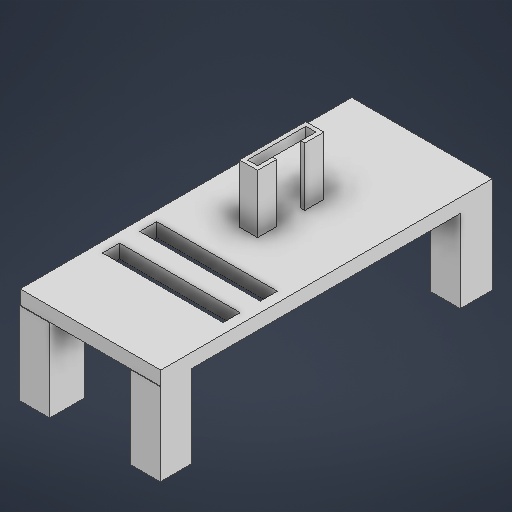
# Autodesk Inventor part: piano laterale
Saved by Autodesk Inventor 2026.2 (Build 302298000, 298)
## iProperties
Created: 2026-01-19
Part Number: piano laterale
Material: Generic
Document SubType Name: Modeling
Designer: ASUS
Density: 1 g/cm^3
Appearance: Default
Mass: 93.3252 g
Surface Area: 462.271 cm^2
Volume: 93.3252 cm^3
Author: ASUS
Autodesk Inventor part; units mm, degrees
ref_plane "YZ Plane" through (0, 0, 0) normal (1, 0, 0) x (0, 1, 0)
ref_plane "XZ Plane" through (0, 0, 0) normal (0, 1, 0) x (-1, 0, 0)
ref_plane "XY Plane" through (0, 0, 0) normal (0, 0, 1) x (1, 0, 0)
sketch "Sketch1" plane through (0, 0, 0) normal (0, 1, 0) x (-1, 0, 0)
  line L0 (0, 0) -> (-70, 0)
  line L1 (-70, 0) -> (-70, 165)
  line L2 (-70, 165) -> (0, 165)
  line L3 (0, 165) -> (0, 0)
  dimension "d0" = 70
  dimension "d1" = 165
  constraints: 8 end point, 2 parallel, 1 horizontal, 1 perpendicular
  measures "d0" distance of L1.end L2.end
  measures "d1" distance of L0.end L1.end
extrude "Extrusion1" add sketch "Sketch1" along normal blind 7
sketch "Sketch2" plane through (0, 0, 0) normal (0, -1, 0) x (1, 0, 0)
  line L0 (70, 165) -> (70, 0) projected
  line L1 (70, 0) -> (55, 0)
  line L2 (55, 0) -> (55, 15.9792)
  line L3 (55, 15.9792) -> (70, 15.9792)
  line L4 (70, 15.9792) -> (70, 0)
  line L5 (70, 0) -> (0, 0) projected
  line L6 (0, 0) -> (15, 0)
  line L7 (15, 0) -> (15, 13.5714)
  line L8 (15, 13.5714) -> (0, 13.5714)
  line L9 (0, 13.5714) -> (0, 0)
  line L10 (70, 165.2646) -> (55, 165.2646)
  line L11 (55, 165.2646) -> (55, 149.7232)
  line L12 (55, 149.7232) -> (70, 149.7232)
  line L13 (70, 149.7232) -> (70, 165.2646)
  line L14 (0, 165.2646) -> (15, 165.2646)
  line L15 (15, 165.2646) -> (15, 148.1909)
  line L16 (15, 148.1909) -> (0, 148.1909)
  line L17 (0, 148.1909) -> (0, 165.2646)
  line L18 (68, 151.7232) -> (57, 151.7232)
  line L19 (57, 151.7232) -> (57, 163.2646)
  line L20 (57, 163.2646) -> (68, 163.2646)
  line L21 (68, 163.2646) -> (68, 151.7232)
  line L22 (2, 150.1909) -> (13, 150.1909)
  line L23 (13, 150.1909) -> (13, 163.2646)
  line L24 (13, 163.2646) -> (2, 163.2646)
  line L25 (2, 163.2646) -> (2, 150.1909)
  line L26 (2, 11.5714) -> (13, 11.5714)
  line L27 (13, 11.5714) -> (13, 2)
  line L28 (13, 2) -> (2, 2)
  line L29 (2, 2) -> (2, 11.5714)
  line L30 (68, 13.9792) -> (57, 13.9792)
  line L31 (57, 13.9792) -> (57, 2)
  line L32 (57, 2) -> (68, 2)
  line L33 (68, 2) -> (68, 13.9792)
  dimension "d4" = 15
  dimension "d5" = 15
  dimension "d6" = 15
  dimension "d7" = 15
  dimension "d8" = 2
  dimension "d9" = 2
  dimension "d10" = 2
  dimension "d11" = 2
  constraints: 64 end point, 16 parallel, 8 perpendicular, 4 horizontal, 3 point on line, 12 other
  measures "d4" distance of L2.end L3.end
  measures "d5" distance of L8.end L7.end
  measures "d6" distance of L12.end L11.end
  measures "d7" distance of L15.end L16.end
  measures "d8" distance between parallel lines of L12 L18
  measures "d9" distance between parallel lines of L16 L22
  measures "d10" distance between parallel lines of L8 L26
  measures "d11" distance between parallel lines of L3 L30
extrude "Extrusion2" add sketch "Sketch2" along normal blind 41
sketch "Sketch3" plane through (0, 7, 0) normal (0, 1, 0) x (1, 0, 0)
  line L0 (18.4911, -158.4869) -> (54.4911, -158.4869) construction
  line L1 (0, -165) -> (70, -165) projected
  line L2 (0, -165) -> (0, -129)
  line L3 (0, -13.5714) -> (0, -148.1909) projected
  line L4 (0, -129) -> (70, -129)
  line L5 (70, -165) -> (70, 0) projected
  line L6 (70, -129) -> (5, -129)
  line L7 (5, -129) -> (5, -120.5)
  line L8 (5, -120.5) -> (70, -120.5)
  line L9 (70, -120.5) -> (70, -129)
  line L10 (70, -110.5) -> (5, -110.5)
  line L11 (5, -110.5) -> (5, -102)
  line L12 (5, -102) -> (70, -102)
  line L13 (70, -102) -> (70, -110.5)
  line L14 (5, -102) -> (65, -102)
  line L15 (65, -182) -> (5, -182)
  line L16 (5, -182) -> (5, -102)
  line L17 (5, -120.5) -> (65, -120.5)
  line L18 (65, -120.5) -> (65, -129)
  line L19 (65, -129) -> (5, -129)
  line L20 (5, -129) -> (5, -120.5)
  line L21 (5, -102) -> (65, -102)
  line L22 (65, -102) -> (65, -110.5)
  line L23 (65, -110.5) -> (5, -110.5)
  line L24 (5, -110.5) -> (5, -102)
  point P0 (0, 0)
  dimension "d16" = 36
  dimension "d17" = 65
  dimension "d18" = 8.5
  dimension "d20" = 65
  dimension "d21" = 8.5
  dimension "d22" = 60
  dimension "d23" = 80
  dimension "d24" = 60
  dimension "d25" = 8.5
  dimension "d26" = 60
  dimension "d27" = 8.5
  constraints: 44 end point, 9 parallel, 6 horizontal, 5 perpendicular, 3 point on line
  measures "d16" distance of L1.start L2.end
  measures "d17" distance of L7.end L8.end
  measures "d18" distance of L6.end L7.end
  measures "d20" distance of L11.end L12.end
  measures "d21" distance of L10.end L11.end
  measures "d22" distance of L15.start L15.end
  measures "d23" distance of L14.end L15.start
  measures "d24" distance of L18.end L19.end
  measures "d25" distance of L17.end L18.end
  measures "d26" distance of L22.end L23.end
  measures "d27" distance of L21.end L22.end
extrude "Extrusion3" cut sketch "Sketch3" against normal blind 7 contours L7 L8 L18 L4 | L11 L12 L22 L10
sketch "Sketch4" plane through (0, 7, 0) normal (0, 1, 0) x (1, 0, 0)
  line L0 (35, -52.8248) -> (30, -52.8248)
  line L1 (30, -52.8248) -> (30, -81.8248)
  line L2 (30, -81.8248) -> (35, -81.8248)
  line L3 (35, -81.8248) -> (35, -52.8248)
  line L4 (37, -50.8248) -> (28, -50.8248)
  line L5 (28, -50.8248) -> (28, -83.8248)
  line L6 (28, -83.8248) -> (37, -83.8248)
  line L7 (37, -83.8248) -> (37, -50.8248)
  point P0 (0, 0)
  dimension "d30" = 5
  dimension "d31" = 29
  dimension "d32" = 2
  constraints: 16 end point, 4 parallel, 2 perpendicular, 1 horizontal, 3 other
  measures "d30" distance of L2.end L1.end
  measures "d31" distance of L1.end L0.end
  measures "d32" distance between parallel lines of L3 L7
extrude "Extrusion4" add sketch "Sketch4" along normal blind 29
sketch "Sketch5" plane through (28, 7, 50.8248) normal (-1, 0, 0) x (0, 0, 1)
  line L0 (2, 0) -> (2, 29) projected
  line L1 (2, 29) -> (2, 0)
  line L2 (31, 0) -> (31, 29) projected
  line L3 (2, 0) -> (31, 0)
  line L4 (31, 0) -> (31, 29)
  line L5 (31, 29) -> (2, 29)
  line L6 (2, 29) -> (31, 29)
  line L7 (31, 29) -> (31, 26)
  line L8 (31, 26) -> (2, 26)
  line L9 (2, 26) -> (2, 29)
  line L10 (2, 26) -> (31, 26)
  line L11 (31, 26) -> (31, 0)
  line L12 (31, 0) -> (2, 0)
  line L13 (2, 0) -> (2, 26)
  point P0 (-50.8248, -7)
  dimension "d35" = 29
  dimension "d36" = 3
  constraints: 24 end point, 6 parallel, 2 horizontal, 2 perpendicular, 1 vertical
  measures "d35" distance of L7.end L8.end
  measures "d36" distance of L6.end L7.end
extrude "Extrusion5" cut sketch "Sketch5" against normal blind 2 contours L0 L8 L2 L3
sketch "Sketch6" plane through (37, 7, 83.8248) normal (1, 0, 0) x (0, 0, -1)
  line L0 (2, 29) -> (31, 29) projected
  line L1 (16.5, 29) -> (16.5, 0)
  line L2 (2, 0) -> (31, 0) projected
  line L3 (23.5, 29) -> (23.5, 0)
  line L4 (9.5, 29) -> (9.5, 0)
  line L5 (9.5, 29) -> (23.5, 29)
  line L6 (23.5, 29) -> (23.5, 0)
  line L7 (23.5, 0) -> (9.5, 0)
  line L8 (9.5, 0) -> (9.5, 29)
  point P0 (83.8248, -7)
  point P1 (23.5, 0)
  point P2 (23.5, 29)
  point P3 (9.5, 29)
  point P4 (9.5, 0)
  dimension "d39" = 7
  dimension "d40" = 7
  constraints: 14 end point, 4 parallel, 2 midpoint, 1 horizontal, 1 perpendicular
  measures "d39" distance between parallel lines of L1 L3
  measures "d40" distance between parallel lines of L1 L4
extrude "Extrusion6" cut sketch "Sketch6" against normal blind 2
sketch "Sketch7" plane through (28, 33, 52.8248) normal (0, -1, 0) x (1, 0, 0)
  line L0 (0, 0) -> (0, 29) projected
  line L1 (2, 29) -> (2, 0) projected
  line L2 (0, 0) -> (2, 0)
  line L3 (2, 0) -> (2, 29)
  line L4 (2, 29) -> (0, 29)
  line L5 (0, 29) -> (0, 0)
  point P0 (-28, -52.8248)
  point P1 (2, 0)
  constraints: 8 end point, 2 parallel, 1 horizontal, 1 perpendicular
extrude "Extrusion7" add sketch "Sketch7" along normal blind 2
body "Solid1"
